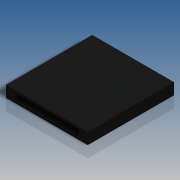
# Autodesk Inventor part: 11034-Black
Saved by Autodesk Inventor 2016 SP2 (Build 200236200, 236)
## iProperties
Created: 2015-08-21
Part Number: 11034-Black
Material: ABS Plastic
Document SubType Name: Modeling
Designer: D. Kohfeld
Mass: 0.258877 g
Surface Area: 9.1328 cm^2
Volume: 0.244224 cm^3
Density: 1.06 g/cm^3
Appearance: Black
Author: D. Kohfeld
Autodesk Inventor part; units mm, degrees
ref_plane "YZ Plane" through (0, 0, 0) normal (1, 0, 0) x (0, 1, 0)
ref_plane "XZ Plane" through (0, 0, 0) normal (0, 1, 0) x (-1, 0, 0)
ref_plane "XY Plane" through (0, 0, 0) normal (0, 0, 1) x (1, 0, 0)
sketch "Sketch2" plane through (0, 0, 0) normal (0, 0, 1) x (1, 0, 0)
  line L0 (-7.2, 1) -> (7.2, 1)
  line L1 (7.2, 1) -> (7.2, -1)
  line L2 (7.2, -1) -> (-7.2, -1)
  line L3 (-7.2, -1) -> (-7.2, 1)
  line L4 (-5.6, 0.6) -> (5.6, 0.6)
  line L5 (5.6, 0.6) -> (5.6, -0.6)
  line L6 (5.6, -0.6) -> (-5.6, -0.6)
  line L7 (-5.6, -0.6) -> (-5.6, 0.6)
  point P0 (0, 0)
  point P1 (-7.2, 0)
  point P2 (0, -1)
  point P3 (0, 0.6)
  point P4 (-5.6, 0)
  dimension "d0" = 2
  dimension "d1" = 14.4
  dimension "d2" = 1.2
  dimension "d3" = 11.2
  constraints: 16 end point, 4 midpoint, 4 parallel, 2 horizontal, 2 horizontal alignment, 2 perpendicular, 2 vertical alignment
  measures "d0" distance of L2.end L0.start
  measures "d1" distance of L0.start L0.end
  measures "d2" distance of L6.end L4.start
  measures "d3" distance of L4.start L4.end
extrude "Extrusion1" add sketch "Sketch2" against normal blind 15.2 contours L0 L1 L2 L3 | L4 L5 L6 L7
extrude "Extrusion2" cut sketch "Sketch2" against normal blind 14.4 contours L4 L5 L6 L7
body "Solid1"
